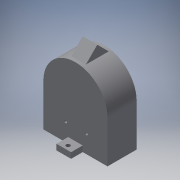
# Autodesk Inventor part: Tail4
Saved by Autodesk Inventor 2016 (Build 200138000, 138)
## iProperties
Created: 2017-03-09
Part Number: Tail4
Material: Generic
Document SubType Name: Modeling
Designer: Owner
Density: 1 g/cm^3
Appearance: Default
Author: Owner
Autodesk Inventor part; units mm, degrees
ref_plane "YZ Plane" through (0, 0, 0) normal (1, 0, 0) x (0, 1, 0)
ref_plane "XZ Plane" through (0, 0, 0) normal (0, 1, 0) x (-1, 0, 0)
sketch "Sketch1" plane through (0, 0, 0) normal (0, 0, 1) x (1, 0, 0)
  line L0 (6.3576, -38.0962) -> (6.3576, -43.1) projected
  line L1 (6.3576, -43.1) -> (22.8752, -43.1) projected
  line L2 (22.8752, -43.1) -> (22.8752, 0) projected
  line L3 (22.8752, 0) -> (22.86, 0) projected
  arc A0 (22.86, 0) -> (-22.86, 0) centre (0, 0) ccw projected
  line L4 (-22.86, 0) -> (-22.86, -43.1) projected
  line L5 (-22.86, -43.1) -> (-6.3424, -43.1) projected
  line L6 (-6.3424, -43.1) -> (-6.3424, -38.0962) projected
  line L7 (-6.3424, -38.0962) -> (6.3576, -38.0962) projected
  line L8 (14.6164, -43.1) -> (-27.9273, -43.1)
  line L9 (-27.9273, -43.1) -> (27.94, -43.1)
  line L10 (0, 0) -> (0, -6.35)
  circle A1 centre (0, -6.35) radius 27.94
  line L11 (-27.94, -6.35) -> (27.94, -6.35)
  line L12 (27.94, -6.35) -> (27.94, -43.1)
  line L13 (27.94, -43.1) -> (-27.94, -43.1)
  line L14 (-27.94, -43.1) -> (-27.94, -6.35)
  point P0 (0, 0)
  dimension "d27" = 55.88
  dimension "d26" = 6.35
  constraints: 14 end point, 2 coincident, 2 parallel, 1 horizontal, 1 horizontal alignment, 1 midpoint, 1 perpendicular, 1 vertical, 2 other
  measures "d26" distance of L10.start L10.end
extrude "Extrusion1" add sketch "Sketch1" along normal blind 25.4 contours L7 L6 L5 L4 A1 L2 L1 L0 | L0 L8 L6 L7 | L2 A1 L12 L9 | L8 L13 L14 A1 L4 | A1 L4 L11 L2 | L2 L11 A1 | A1 L11 L4 | L11 L4 A0 A1 L3 L2 | L2 L3 A0 A1 L11 | L11 A1 A0 L4
sketch "Sketch2" plane through (0, 0, 0) normal (0, 0, -1) x (-1, 0, 0)
  line L0 (7.62, -43.1) -> (-7.62, -43.1) projected
  line L1 (-7.62, -43.1) -> (-7.62, -38.0962) projected
  line L2 (-7.62, -38.0962) -> (7.62, -38.0962) projected
  line L3 (7.62, -38.0962) -> (7.62, -43.1) projected
  line L4 (-0.0064, -43.1) -> (6.3436, -43.1)
  line L5 (6.3436, -43.1) -> (-6.3564, -43.1)
  line L6 (6.3436, -43.1) -> (-6.35, -43.1)
  line L7 (-6.35, -38.0962) -> (6.35, -38.0962)
  line L8 (-6.35, -38.0962) -> (6.35, -38.0962)
  line L9 (6.35, -38.0962) -> (6.35, -33.0924)
  line L10 (6.35, -33.0924) -> (-6.35, -33.0924)
  line L11 (-6.35, -33.0924) -> (-6.35, -38.0962)
  point P0 (0, 0)
  dimension "d19" = 6.35
  dimension "d20" = 12.7
  dimension "d21" = 5.0038
  constraints: 16 end point, 3 parallel, 2 horizontal, 1 perpendicular
  measures "d19" distance of L4.start L4.end
  measures "d20" distance of L4.end L5.end
  measures "d21" distance of L10.end L7.start
extrude "Extrusion2" add sketch "Sketch2" along normal blind 10.16 contours L2 L11 L10 L9
sketch "Sketch4" plane through (0, 0, 25.4) normal (0, 0, 1) x (1, 0, 0)
  line L0 (0.0064, -43.1) -> (6.3564, -43.1)
  line L1 (6.3564, -43.1) -> (-6.3436, -43.1)
  line L2 (-6.3436, -43.1) -> (6.35, -43.1)
  line L3 (6.35, -43.1) -> (6.35, -38.0962)
  line L4 (6.35, -38.0962) -> (-6.3436, -38.0962)
  line L5 (-6.3436, -38.0962) -> (-6.3436, -43.1)
  point P0 (0, 0)
  dimension "d10" = 6.35
  dimension "d11" = 12.7
  dimension "d12" = 5.0038
  constraints: 12 end point, 2 parallel, 1 horizontal, 1 perpendicular
  measures "d10" distance of L0.start L0.end
  measures "d11" distance of L0.end L1.end
  measures "d12" distance of L2.end L3.end
extrude "Extrusion4" add sketch "Sketch4" along normal blind 10.16
sketch "Sketch5" plane through (-6.3436, -38.0962, 25.4) normal (0, 1, 0) x (1, 0, 0)
  line L0 (12.6936, -10.16) -> (0, -10.16) projected
  line L1 (6.3468, -10.16) -> (6.3468, -6.35)
  circle A0 centre (6.3468, -6.35) radius 1.75
  point P0 (6.3436, 25.4)
  dimension "d15" = 3.81
  dimension "d16" = 3.5
  constraints: 2 end point, 1 centre point, 1 coincident, 1 midpoint, 1 vertical
  measures "d15" distance of L1.start L1.end
  measures "d16" diameter of A0
extrude "Extrusion5" cut sketch "Sketch5" against normal blind 10.16
sketch "Sketch6" plane through (-6.35, -33.0924, 0) normal (0, 1, 0) x (1, 0, 0)
  line L0 (12.7, 10.16) -> (0, 10.16) projected
  line L1 (6.35, 10.16) -> (6.35, 6.35)
  circle A0 centre (6.35, 6.35) radius 2.25
  point P0 (6.35, 0)
  dimension "d22" = 3.81
  dimension "d23" = 4.5
  constraints: 2 end point, 1 centre point, 1 coincident, 1 midpoint, 1 vertical
  measures "d22" distance of L1.start L1.end
  measures "d23" diameter of A0
extrude "Extrusion6" cut sketch "Sketch6" against normal blind 10.16
ref_plane "Work Plane1" through (0, -43.1, 0) normal (-1, 0, 0) x (0, 0, 1)
sketch "Sketch7" plane through (0, -43.1, 0) normal (-1, 0, 0) x (0, 0, 1)
  line L0 (0, 64.69) -> (0, 36.75) projected
  line L1 (0, 64.69) -> (2.7051, 64.69)
  line L2 (0, 64.69) -> (25.4, 64.69) projected
  line L3 (2.7051, 64.69) -> (22.6949, 64.69)
  line L4 (22.6949, 64.69) -> (12.6873, 64.69)
  line L5 (12.6873, 64.69) -> (12.6873, 74.6976)
  line L6 (12.6873, 74.6976) -> (22.6949, 64.69)
  line L7 (12.6873, 74.6976) -> (2.7051, 64.69)
  point P0 (0, 43.1)
  dimension "d29" = 2.7051
  dimension "d30" = 19.9898
  dimension "d31" = 10.0076
  dimension "d32" = 10.0076
  constraints: 12 end point, 3 point on line, 1 perpendicular
  measures "d29" distance of L0.start L1.end
  measures "d30" distance of L1.end L3.end
  measures "d31" distance of L3.end L4.end
  measures "d32" distance of L4.end L5.end
extrude "Extrusion7" add sketch "Sketch7" along normal mid plane 12.7
sketch "Sketch8" plane through (0, 0, 0) normal (0, 0, -1) x (-1, 0, 0)
  ellipse E0 centre (-10.537, -27.5683) end of major axis (-10.537, -26.3183) minor radius 1.25 projected
  ellipse E1 centre (9.593, -27.5683) end of major axis (9.593, -26.3237) minor radius 1.2446 projected
  line L0 (-10.537, -27.5683) -> (-9.537, -27.5683)
  line L1 (9.593, -27.5683) -> (8.593, -27.5683)
  circle A0 centre (-9.537, -27.5683) radius 1.2446
  circle A1 centre (8.593, -27.5683) radius 1.2446
  point P0 (0, 0)
  dimension "d35" = 1
  dimension "d36" = 1
  dimension "d37" = 2.4892
  dimension "d38" = 2.4892
  constraints: 4 end point, 2 centre point, 2 coincident, 2 horizontal, 2 other
  measures "d35" distance of L0.start L0.end
  measures "d36" distance of L1.start L1.end
  measures "d37" diameter of A0
  measures "d38" diameter of A1
extrude "Extrusion8" cut sketch "Sketch8" against normal blind 25.4 contours A0 E0 | E0 A0 | A1 E1 | E1 A1 picked at (-10.2799, -27.7436) picked at (-8.6366, -27.4668) picked at (9.3378, -27.743) picked at (7.6944, -27.4665)
body "Solid1"
